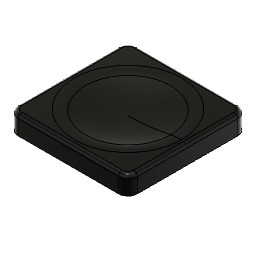
keycap v16 (Autodesk Fusion 360 design; units mm, degrees)
Autodesk Fusion 360 part; units mm, degrees
sketch "plan" plane through (0, 0, 0) normal (0, 1, 0) x (1, 0, 0)
  line L0 (8, 8) -> (-8, 8)
  line L1 (-8, 8) -> (-8, -8)
  line L2 (-8, -8) -> (8, -8)
  line L3 (8, -8) -> (8, 8)
  line L4 (7, 7) -> (-7, 7)
  line L5 (-7, 7) -> (-7, -7)
  line L6 (-7, -7) -> (7, -7)
  line L7 (7, -7) -> (7, 7)
  line L8 (-3.48, 0) -> (3.48, 0) construction
  line L9 (-3.48, -1.48) -> (-2.2, -1.48)
  line L10 (-2.2, -1.48) -> (-2.2, 1.48)
  line L11 (-2.2, 1.48) -> (-3.48, 1.48)
  line L12 (-3.48, 1.48) -> (-3.48, -1.48)
  line L13 (-7, 7) -> (7, -7) construction
  line L14 (-8, -8) -> (8, 8) construction
  line L15 (2.2, -1.48) -> (3.48, -1.48)
  line L16 (3.48, -1.48) -> (3.48, 1.48)
  line L17 (3.48, 1.48) -> (2.2, 1.48)
  line L18 (2.2, 1.48) -> (2.2, -1.48)
  dimension "d1" = 16
  dimension "d2" = 16
  dimension "d3" = 1
  dimension "d5" = 1
  dimension "d10" = 6.96
  dimension "d11" = 1.28
  dimension "d12" = 2.96
  dimension "d13" = 1.28
  dimension "d14" = 2.96
  constraint horizontal L0
  constraint horizontal L4
  constraint midpoint origin L8
  constraint horizontal L8
  constraint horizontal L9
  constraint vertical L10
  constraint horizontal L11
  constraint vertical L12
  constraint midpoint L8.start L12
  constraint horizontal L6
  constraint horizontal L2
  constraint vertical L7
  constraint vertical L3
  constraint vertical L5
  constraint midpoint origin L13
  constraint midpoint L13 L14
  constraint horizontal L15
  constraint vertical L16
  constraint horizontal L17
  constraint vertical L18
  constraint midpoint L8.end L16
  measures "d1" distance of L1.end L2.end
  measures "d2" distance of L0.end L1.end
  measures "d3" distance of L0 L4
  measures "d5" distance of L1 L5
  measures "d10" horizontal distance of L8.start L8.end
  measures "d11" distance of L9.start L9.end
  measures "d12" distance of L9 L11
  measures "d13" distance of L15.start L15.end
  measures "d14" distance of L15.end L16.end
extrude "Extrude1" add sketch "plan" along normal blind 1.5 contours L0 L1 L2 L3 | L4 L5 L6 L7 | L9 L10 L11 L12 | L15 L16 L17 L18
extrude "Extrude2" add sketch "plan" against normal blind 1 contours L0 L1 L2 L3
extrude "Extrude3" add sketch "plan" against normal blind 2.96 contours L9 L10 L11 L12 | L15 L16 L17 L18
sketch "indent" plane through (0, 0, 0) normal (0, 0, 1) x (1, 0, 0)
  line L0 (8, -1) -> (8, 1.5)
  line L1 (8, 1.5) -> (8, -1)
  line L2 (8, 1.5) -> (-8, 1.5)
  line L3 (-8, 1.5) -> (8, 1.5)
  line L4 (-8, -1) -> (-8, 1.5)
  line L5 (-8, 1.5) -> (-8, -1)
  line L6 (-8, 0) -> (8, 0)
  line L7 (0, 1.5) -> (0, 0.7)
  spline S0 degree 5 poles (-6.4, 1.5) (-6.144, 1.4393) (-5.632, 1.3233) (-4.864, 1.1651) (-3.84, 0.9865) (-2.56, 0.8208) (-1.28, 0.7177) (0, 0.6824) (1.28, 0.7177) (2.56, 0.8208) (3.84, 0.9865) (4.864, 1.1651) (5.632, 1.3233) (6.144, 1.4393) (6.4, 1.5) knots 0 0 0 0 0 0 0.1 0.2 0.3 0.4 0.5 0.6 0.7 0.8 0.9 1 1 1 1 1 1
  point P0 (-8, 0)
  point P1 (8, 0)
  point P2 (-6.4, 1.5)
  point P3 (6.4, 1.5)
  dimension "d17" = 1.6
  dimension "d18" = 1.6
  dimension "d20" = 0.8
  constraint coincident P0 L6.start
  constraint coincident P1 L6.end
  constraint midpoint L2 L7.start
  constraint vertical L7
  constraint coincident L3 P2
  constraint coincident L3 P3
  constraint coincident P2 S0.start
  constraint coincident P3 S0.end
  measures "d17" distance of L2.end P2
  measures "d18" distance of L0.end S0.end
  measures "d20" distance of L7.start L7.end
revolve "Revolve1" cut sketch "indent" angle 360 about axis through (0, 1.75, 0) along (0, 1, 0) contours L2 L3 L7 S0 picked at (0.7111, 0.9984)
fillet "Fillet1" radius 1.25 4 edges at (-8, 0.25, 8) (8, 0.25, 8) (8, 0.25, -8) (-8, 0.25, -8)
fillet "Fillet2" radius 0.5 8 edges at (7.6339, 1.5, -7.6339) (0, 1.5, -8) (-7.6339, 1.5, -7.6339) (-8, 1.5, 0) (-7.6339, 1.5, 7.6339) (0, 1.5, 8) (7.6339, 1.5, 7.6339) (8, 1.5, 0)
fillet "Fillet3" radius 7 1 edges at (-5.9669, 1.5, -2.3143)
equation "d13 = d11"
equation "d14 = d12"
equation "d18 = d17"
